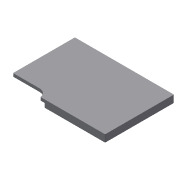
# Autodesk Inventor part: Boden
Saved by Autodesk Inventor 2020 (Build 240168000, 168)
## iProperties
Created: 2022-10-11
Part Number: Boden
Material: Allgemein
Document SubType Name: Modeling
Designer: uch10113
Density: 1 g/cm^3
Appearance: Vorgabe
Author: uch10113
Autodesk Inventor part; units mm, degrees
ref_plane "YZ Plane" through (0, 0, 0) normal (1, 0, 0) x (0, 1, 0)
ref_plane "XZ Plane" through (0, 0, 0) normal (0, 1, 0) x (-1, 0, 0)
ref_plane "XY Plane" through (0, 0, 0) normal (0, 0, 1) x (1, 0, 0)
sketch "Skizze1" plane through (0, 0, 0) normal (0, 0, 1) x (1, 0, 0)
  line L0 (-7.1596, -18.5) -> (23.8404, -18.5) projected
  arc A0 (23.8404, -18.5) -> (25.8404, -16.5) centre (23.8404, -16.5) ccw projected
  line L1 (25.8404, -16.5) -> (25.8404, 16.5) projected
  arc A1 (25.8404, 16.5) -> (23.8404, 18.5) centre (23.8404, 16.5) ccw projected
  line L2 (23.8404, 18.5) -> (-23.8404, 18.5) projected
  arc A2 (-23.8404, 18.5) -> (-25.8404, 16.5) centre (-23.8404, 16.5) ccw projected
  line L3 (-25.8404, 16.5) -> (-25.8404, -13.1) projected
  arc A3 (-25.8404, -13.1) -> (-23.8404, -15.1) centre (-23.8404, -13.1) ccw projected
  line L4 (-23.8404, -15.1) -> (-11.1143, -15.1) projected
  arc A4 (-9.1369, -16.8) -> (-11.1143, -15.1) centre (-11.1143, -17.1) ccw projected
  arc A5 (-9.1369, -16.8) -> (-7.1596, -18.5) centre (-7.1596, -16.5) ccw projected
  line L5 (-24.3404, -13.1) -> (-24.3404, 16.5) projected
  arc A6 (-23.8404, 17) -> (-24.3404, 16.5) centre (-23.8404, 16.5) ccw projected
  line L6 (-23.8404, 17) -> (23.8404, 17) projected
  arc A7 (24.3404, 16.5) -> (23.8404, 17) centre (23.8404, 16.5) ccw projected
  line L7 (24.3404, 16.5) -> (24.3404, -16.5) projected
  arc A8 (23.8404, -17) -> (24.3404, -16.5) centre (23.8404, -16.5) ccw projected
  line L8 (23.8404, -17) -> (-7.1596, -17) projected
  arc A9 (-7.6539, -16.575) -> (-7.1596, -17) centre (-7.1596, -16.5) ccw projected
  arc A10 (-7.6539, -16.575) -> (-11.1143, -13.6) centre (-11.1143, -17.1) ccw projected
  line L9 (-11.1143, -13.6) -> (-23.8404, -13.6) projected
  arc A11 (-24.3404, -13.1) -> (-23.8404, -13.6) centre (-23.8404, -13.1) ccw projected
  line L10 (23.8404, 16.7) -> (-23.8404, 16.7)
  arc A12 (-23.8404, 16.7) -> (-24.0404, 16.5) centre (-23.8404, 16.5) ccw
  line L11 (-24.0404, 16.5) -> (-24.0404, -13.1)
  arc A13 (-24.0404, -13.1) -> (-23.8404, -13.3) centre (-23.8404, -13.1) ccw
  line L12 (-23.8404, -13.3) -> (-11.1143, -13.3)
  arc A14 (-7.3573, -16.53) -> (-11.1143, -13.3) centre (-11.1143, -17.1) ccw
  arc A15 (-7.3573, -16.53) -> (-7.1596, -16.7) centre (-7.1596, -16.5) ccw
  line L13 (-7.1596, -16.7) -> (23.8404, -16.7)
  arc A16 (23.8404, -16.7) -> (24.0404, -16.5) centre (23.8404, -16.5) ccw
  line L14 (24.0404, -16.5) -> (24.0404, 16.5)
  arc A17 (24.0404, 16.5) -> (23.8404, 16.7) centre (23.8404, 16.5) ccw
  point P0 (0, 0)
  dimension "d0" = 0.3
  constraints: 12 point on circle, 10 end point, 6 centre point, 10 other
  measures "d0" distance between parallel lines of L6 L10
extrude "Extrusion1" add sketch "Skizze1" against normal blind 1.5 contours A17 L14 A16 L13 A15 A14 L12 A13 L11 A12 L10
sketch "Skizze2" plane through (0, 0, -1.5) normal (0, 0, -1) x (-1, 0, 0)
  line L0 (6.2404, -13.1) -> (6.2404, 16.5) projected
  arc A0 (11.1143, -13.3) -> (7.3573, -16.53) centre (11.1143, -17.1) ccw projected
  arc A1 (7.1596, -16.7) -> (7.3573, -16.53) centre (7.1596, -16.5) ccw projected
  line L1 (7.1596, -16.7) -> (-23.8404, -16.7) projected
  arc A2 (-24.0404, -16.5) -> (-23.8404, -16.7) centre (-23.8404, -16.5) ccw projected
  line L2 (-24.0404, -16.5) -> (-24.0404, 16.5) projected
  arc A3 (-23.8404, 16.7) -> (-24.0404, 16.5) centre (-23.8404, 16.5) ccw projected
  line L3 (-23.8404, 16.7) -> (23.8404, 16.7) projected
  arc A4 (24.0404, 16.5) -> (23.8404, 16.7) centre (23.8404, 16.5) ccw projected
  line L4 (24.0404, 16.5) -> (24.0404, -13.1) projected
  arc A5 (23.8404, -13.3) -> (24.0404, -13.1) centre (23.8404, -13.1) ccw projected
  line L5 (23.8404, -13.3) -> (11.1143, -13.3) projected
  line L6 (5.2404, -37.9441) -> (-28.2922, -37.9441)
  line L7 (-28.2922, -37.9441) -> (-28.2922, 30.637)
  line L8 (-28.2922, 30.637) -> (5.2404, 30.637)
  line L9 (5.2404, 30.637) -> (5.2404, -37.9441)
  point P0 (0, 0)
  point P1 (5.2404, -16.7)
  point P2 (5.2404, 16.7)
  dimension "d3" = 1
  constraints: 8 end point, 2 parallel, 1 horizontal, 1 perpendicular
  measures "d3" distance between parallel lines of L0 L9
extrude "Extrusion2" add sketch "Skizze2" along normal blind 3 contours L1 A2 L2 A3 L3 L9
sketch "Skizze3" plane through (-7.1596, -16.7, 0) normal (0, -1, 0) x (1, 0, 0)
  circle A0 centre (28, -3) radius 2 projected
  circle A1 centre (4, -3) radius 2 projected
  circle A2 centre (28, -3) radius 0.9
  circle A3 centre (4, -3) radius 0.9
  point P0 (7.1596, 0)
  dimension "d6" = 1.8
  dimension "d7" = 1.8
  constraints: 2 centre point, 2 coincident
  measures "d6" diameter of A2
  measures "d7" diameter of A3
extrude "Extrusion3" cut sketch "Skizze3" against normal through all contours A2 | A3
chamfer "Fase1" distance 0.5 angle 45 4 edges at (-4.0596, 16.7, -3) (19.9404, 16.7, -3) (19.9404, -16.7, -3) (-4.0596, -16.7, -3)
